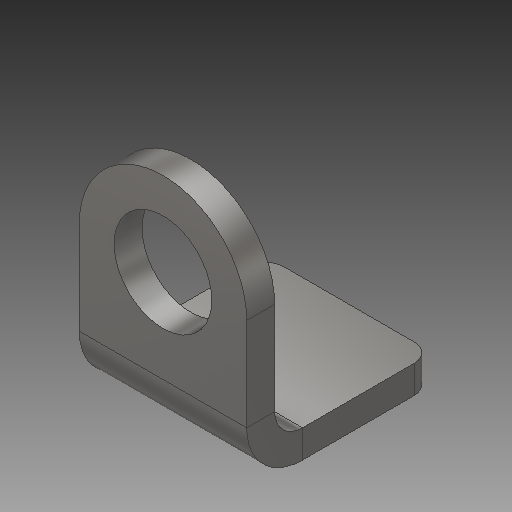
# Autodesk Inventor part: Supporto perno tendi motore
Saved by Autodesk Inventor 2018 (Build 220112000, 112)
## iProperties
Created: 2020-06-04
Part Number: Supporto perno tendi motore
Material: Acciaio inossidabile
Document SubType Name: Lamiera
Designer: Francesco
Density: 8 g/cm^3
Sheet Metal Rule: Default_mm
Appearance: Semilucidato
Mass: 14.3559 g
Surface Area: 16.1537 cm^2
Volume: 1.79449 cm^3
Author: Francesco
Autodesk Inventor part; units mm, degrees
ref_plane "YZ Plane" through (0, 0, 0) normal (1, 0, 0) x (0, 1, 0)
ref_plane "XZ Plane" through (0, 0, 0) normal (0, 1, 0) x (-1, 0, 0)
ref_plane "XY Plane" through (0, 0, 0) normal (0, 0, 1) x (1, 0, 0)
sketch "Schizzo1" plane through (0, 0, 0) normal (0, 0, 1) x (1, 0, 0)
  circle A0 centre (0, 0) radius 5.25
  arc A1 (9, 0) -> (-9, 0) centre (0, 0) ccw
  line L0 (-9, 0) -> (-9, -10)
  line L1 (-9, -10) -> (9, -10)
  line L2 (9, -10) -> (9, 0)
  dimension "d0" = 10.5
  dimension "d1" = 18
  dimension "d2" = 10
  measures "d0" diameter of A0
  measures "d1" diameter of A1
  measures "d2" distance of L0.start L0.end
extrude "Piano1" add sketch "Schizzo1" along normal blind 3
sketch "Schizzo2" plane through (-9, -13, -3) normal (0, -1, 0) x (1, 0, 0)
  line L0 (18, 0) -> (0, 0)
  line L1 (0, 0) -> (0, -14)
  line L2 (0, -14) -> (18, -14)
  line L3 (18, -14) -> (18, 0)
  constraints: 6 end point, 1 horizontal, 1 perpendicular, 1 vertical
edge flange "Flangia1" height 20 angle 90 thickness 3 bend radius 3 thickness toward (0, -1, 0) relief tear relief width 3 relief depth 1.5 edges at (0, -10, 0) wall of the first edge with corners at (9, -13, -3) (-9, -13, -3) (-9, -13, -17) (9, -13, -17)
bend "Piega (Bend)1"
corner "Angolo1"
fillet "Arrotondamento angolo1" radius 2 2 edges at (9, -14.5, -17) (-9, -14.5, -17)
equation "\"d3\" = Spessore"
equation "\"d4\" = LarghezzaScaricoPiega"
equation "\"d5\" = ProfonditàScaricoPiega"
equation "\"d6\" = ResiduoMinimo"
equation "\"d7\" = RaggioTransizione"
equation "\"d10\" = RaggioPiega"
equation "\"d11\" = DimensioniScaricoAngolo"
equation "\"d12\" = DimensioneGioco"
equation "\"d13\" = Dimensione_raggio_Jacobi"
equation "\"RaggioPiega\" = Spessore"
equation "\"LarghezzaScaricoPiega\" = Spessore"
equation "\"ProfonditàScaricoPiega\" = 0.5 * Spessore"
equation "\"DimensioniScaricoAngolo\" = 4 * Spessore"
equation "\"ResiduoMinimo\" = 2 * Spessore"
equation "\"RaggioTransizione\" = RaggioPiega"
equation "\"Dimensione_raggio_Jacobi\" = RaggioPiega"
equation "\"DimensioneGioco\" = Spessore"
equation "\"Spessore\" = 3"
